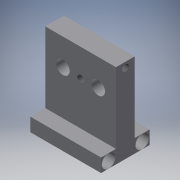
# Autodesk Inventor part: coulissant coté
Saved by Autodesk Inventor 2017 (Build 210142000, 142)
## iProperties
Created: 2018-11-10
Part Number: coulissant coté
Material: Generic
Document SubType Name: Modeling
Designer: Antoine Blaud
Density: 1 g/cm^3
Appearance: Default
Author: Antoine Blaud
Autodesk Inventor part; units mm, degrees
ref_plane "YZ Plane" through (0, 0, 0) normal (1, 0, 0) x (0, 1, 0)
ref_plane "XZ Plane" through (0, 0, 0) normal (0, 1, 0) x (-1, 0, 0)
ref_plane "XY Plane" through (0, 0, 0) normal (0, 0, 1) x (1, 0, 0)
sketch "Sketch2" plane through (0, 0, 0) normal (1, 0, 0) x (0, 1, 0)
  circle A0 centre (0, 0) radius 3.81
  line L0 (-3.81, 4.2173) -> (3.81, 4.2173)
  line L1 (3.81, 4.2173) -> (3.81, -4.2173)
  line L2 (3.81, -4.2173) -> (-3.81, -4.2173)
  line L3 (-3.81, -4.2173) -> (-3.81, 4.2173)
  line L4 (-3.81, 4.2173) -> (3.81, -4.2173) construction
  line L5 (3.81, 4.2173) -> (-3.81, -4.2173) construction
  circle A1 centre (0, 19.05) radius 3.81
  line L6 (-3.81, 23.2673) -> (3.81, 23.2673)
  line L7 (3.81, 23.2673) -> (3.81, 14.8327)
  line L8 (3.81, 14.8327) -> (-3.81, 14.8327)
  line L9 (-3.81, 14.8327) -> (-3.81, 23.2673)
  line L10 (-3.81, 23.2673) -> (3.81, 14.8327) construction
  line L11 (3.81, 23.2673) -> (-3.81, 14.8327) construction
  line L12 (0, 0) -> (0, 19.05)
  line L13 (-3.81, 14.8327) -> (-3.81, 4.2173)
  line L14 (3.81, 14.8327) -> (3.81, 4.2173)
  line L15 (3.81, 14.8327) -> (43.81, 14.8327)
  line L16 (43.81, 14.8327) -> (43.81, 4.2173)
  line L17 (43.81, 4.2173) -> (3.81, 4.2173)
  dimension "d42" = 7.62
  dimension "d43" = 42.096
  dimension "d46" = 7.62
  dimension "d47" = 42.096
  dimension "d48" = 19.05
  dimension "d49" = 40
  constraints: 36 end point, 4 midpoint, 4 parallel, 4 perpendicular, 2 centre point, 2 coincident, 2 horizontal, 2 tangent, 1 point on line, 1 vertical
  measures "d42" diameter of A0
  measures "d43" angle of L4 L1
  measures "d46" diameter of A1
  measures "d47" angle of L10 L7
  measures "d48" distance of point (0, 19.05) point (0, 0)
  measures "d49" distance between parallel lines of L16 L7
extrude "Extrusion6" add sketch "Sketch2" along normal blind 40 contours L1 L2 L3 A0 | A0 L12 L0 L1 | A0 L3 L0 L12 | L0 L12 L8 L14 | L14 L15 L16 L17 | L0 L13 L8 L12 | L8 L12 A1 L7 | L8 L9 A1 L12 | A1 L9 L6 L7
sketch "Sketch3" plane through (0, 3.81, 4.2173) normal (0, 0, -1) x (-1, 0, 0)
  line L0 (0, 40) -> (-40, 40) projected
  line L1 (0, 0) -> (0, 40) projected
  line L2 (-40, 40) -> (0, 40)
  line L3 (0, 40) -> (0, 0)
  line L4 (0, 0) -> (-40, 0)
  line L5 (-40, 0) -> (-40, 40)
  line L6 (-40, 40) -> (0, 0)
  line L7 (0, 0) -> (-40, 0) projected
  line L8 (-40, 0) -> (0, 40)
  line L9 (-20, 30) -> (-40, 20)
  line L10 (-40, 0) -> (-40, 40) projected
  line L11 (-20, 30) -> (0, 20)
  circle A0 centre (-30, 25) radius 3.81
  circle A1 centre (-10, 25) radius 3.81
  line L12 (-20, 40) -> (-20, 0)
  line L13 (0, 0) -> (-40, 0) projected
  circle A2 centre (-20, 24.4225) radius 1.905
  point P0 (0, -3.81)
  dimension "d51" = 10
  dimension "d52" = 20
  dimension "d55" = 7.62
  dimension "d56" = 7.62
  dimension "d57" = 3.81
  dimension "d58" = 15.5776
  constraints: 18 end point, 6 midpoint, 3 centre point, 3 coincident, 2 parallel, 1 horizontal, 1 perpendicular, 1 point on line
  measures "d51" distance from line of L9.start L0
  measures "d52" distance from line of L9.start L1
  measures "d55" diameter of A0
  measures "d56" diameter of A1
  measures "d57" diameter of A2
  measures "d58" distance from line of point (-20, 24.422) L0
extrude "Extrusion7" cut sketch "Sketch3" against normal blind 40 contours A1 L11 L8 | L8 L11 A1 | A1 L8 L11 | L8 A1 L11 | A0 L9 L6 | L6 L9 A0 | A0 L6 L9 | A2 L12 | L12 A2 | L9 L6 A0
thread "Thread6" size "M1x0.25" class "6H" standard "ISO Metric profile" full length
sketch "Sketch4" plane through (40, 0, 0) normal (1, 0, 0) x (0, 0, -1)
  line L0 (-14.8327, 3.81) -> (-4.2173, 3.81)
  line L1 (-4.2173, 3.81) -> (-4.2173, 43.81)
  line L2 (-4.2173, 43.81) -> (-14.8327, 43.81)
  line L3 (-14.8327, 43.81) -> (-14.8327, 3.81)
  line L4 (-9.525, 3.81) -> (-9.525, 43.81)
  circle A0 centre (-9.525, 40.7005) radius 1.905
  point P0 (0, 0)
  point P1 (-9.525, 13.81)
  dimension "d61" = 3.81
  constraints: 10 end point, 2 midpoint, 2 parallel, 1 centre point, 1 horizontal, 1 perpendicular, 1 point on line
  measures "d61" diameter of A0
extrude "Extrusion8" cut sketch "Sketch4" against normal blind 150 contours A0 L4 | L4 A0
thread "Thread7" size "M1x0.25" class "6H" standard "ISO Metric profile" full length
body "Solid3"
